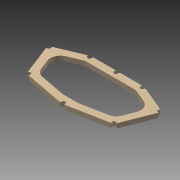
# Autodesk Inventor part: section1
Saved by Autodesk Inventor 2015 (Build 190159000, 159)
## iProperties
Created: 2017-09-23
Part Number: section1
Material: Polyethylene, High Density
Document SubType Name: Modeling
Designer: Mimoja
Density: 0.952 g/cm^3
Appearance: Smooth - Off-White
Mass: 481.217 g
Surface Area: 933.765 cm^2
Volume: 505.48 cm^3
Author: Mimoja
Autodesk Inventor part; units mm, degrees
ref_plane "YZ Plane" through (0, 0, 0) normal (1, 0, 0) x (0, 1, 0)
ref_plane "XZ Plane" through (0, 0, 0) normal (0, 1, 0) x (-1, 0, 0)
ref_plane "XY Plane" through (0, 0, 0) normal (0, 0, 1) x (1, 0, 0)
sketch "Sketch1" plane through (0, 0, 0) normal (0, 0, 1) x (1, 0, 0)
  line L0 (0, 8.2296) -> (-172.5168, 41.148)
  line L1 (-172.5168, 41.148) -> (-225.8568, 178.0032)
  line L2 (-225.8568, 178.0032) -> (-105.7656, 228.6)
  line L3 (0, 569.8709) -> (0, -138.2601) construction
  line L4 (-105.7656, 228.6) -> (0, 228.6)
  line L5 (0, 228.6) -> (0, 8.2296)
  point P0 (0, 0)
  dimension "d9" = 228.6
  dimension "d11" = 225.8568
  dimension "d15" = 178.0032
  dimension "d20" = 172.5168
  dimension "d22" = 41.148
  dimension "d39" = 105.7656
  dimension "d41" = 0
  dimension "d42" = 8.2296
  constraints: 12 end point, 1 collinear, 1 perpendicular, 1 point on line, 1 vertical
  measures "d9" vertical distance of point (0, 0) L2.end
  measures "d11" horizontal distance of point (0, 0) L1.end
  measures "d15" vertical distance of point (0, 0) L1.end
  measures "d20" horizontal distance of point (0, 0) L0.end
  measures "d22" vertical distance of point (0, 0) L0.end
  measures "d39" horizontal distance of point (0, 0) L2.end
  measures "d41" horizontal distance of point (0, 0) L0.start
  measures "d42" distance of point (0, 0) L0.start
extrude "Extrusion4" add sketch "Sketch1" along normal blind 18
hole "Hole2" at (0.0182, 221.5256, 18) direction (0, 0, -1) diameter 15 end through all
hole "Hole3" at (-219.4433, 175.7937, 18) direction (0, 0, -1) diameter 15 end through all
hole "Hole4" at (-168.4127, 45.8852, 18) direction (0, 0, -1) diameter 15 end through all
hole "Hole5" at (0.2097, 14.8483, 18) direction (0, 0, -1) diameter 15 end through all
hole "Hole6" at (-104.4112, 221.9476, 18) direction (0, 0, -1) diameter 15 end through all
fillet "Fillet6" radius 4 1 edges at (-2.4724, 228.6, 9)
fillet "Fillet7" radius 3 1 edges at (-100.9477, 228.6, 9)
fillet "Fillet8" radius 3 1 edges at (-110.1804, 226.74, 9)
fillet "Fillet9" radius 1 1 edges at (-215.6897, 182.2868, 9)
fillet "Fillet10" radius 1 1 edges at (-222.2915, 168.8555, 9)
fillet "Fillet11" radius 1 1 edges at (-175.4126, 48.5779, 9)
fillet "Fillet12" radius 1 1 edges at (-164.3395, 39.5877, 9)
fillet "Fillet13" radius 3 1 edges at (-4.6212, 9.1114, 9)
sketch "Sketch4" plane through (0, 0, 18) normal (0, 0, 1) x (1, 0, 0)
  line L0 (0, 200.6) -> (-100.1079, 200.6)
  line L1 (-100.1079, 200.6) -> (-189.8721, 162.7806)
  line L2 (-11.0632, 228.6) -> (-94.5669, 228.6) projected
  line L3 (-116.0663, 224.2601) -> (-214.0734, 182.9678) projected
  line L4 (-189.8721, 162.7806) -> (-152.0534, 65.7485)
  line L5 (-152.0534, 65.7485) -> (-30, 42.4592)
  line L6 (-30, 42.4592) -> (0, 42.4592)
  line L7 (0, 22.3454) -> (0, 214.0256) projected
  line L8 (-221.5743, 167.0156) -> (-176.187, 50.5648) projected
  line L9 (-162.2988, 39.1983) -> (-10.7261, 10.2763) projected
  line L10 (0, 200.6) -> (0, 42.4592)
  dimension "d175" = 30
  dimension "d176" = 28
  dimension "d177" = 28
  dimension "d178" = 28
  dimension "d179" = 28
  constraints: 12 end point, 4 parallel, 1 collinear, 1 horizontal, 1 point on line
  measures "d175" distance of L5.end L6.end
  measures "d176" distance between parallel lines of L8 L4
  measures "d177" distance between parallel lines of L3 L1
  measures "d178" distance between parallel lines of L2 L0
  measures "d179" distance between parallel lines of L9 L5
extrude "Extrusion5" cut sketch "Sketch4" against normal through all
fillet "Fillet14" radius 40 4 edges at (-152.0534, 65.7485, 9) (-189.8721, 162.7806, 9) (-100.1079, 200.6, 9) (-30, 42.4592, 9)
mirror "Mirror3" about plane through (0, 0, 0) normal (1, 0, 0)
body "Solid4"
